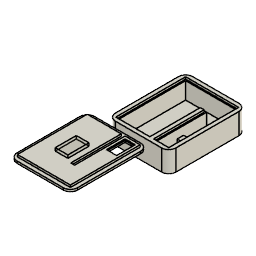
modelo_v2 (Autodesk Fusion 360 design; units mm, degrees)
part number: 2026-04-27-17-29-00-907
Autodesk Fusion 360 part; units mm, degrees
sketch "Boceto1" plane through (0, 0, 0) normal (0, 0, 1) x (1, 0, 0)
  line L0 (115, 170) -> (5, 170)
  arc A0 (5, 170) -> (-10, 155) centre (5, 155) ccw
  line L1 (-10, 155) -> (-10, 5)
  arc A1 (-10, 5) -> (5, -10) centre (5, 5) ccw
  line L2 (5, -10) -> (115, -10)
  arc A2 (115, -10) -> (130, 5) centre (115, 5) ccw
  line L3 (130, 5) -> (130, 155)
  arc A3 (130, 155) -> (115, 170) centre (115, 155) ccw
  line L4 (115, 170) -> (5, 170)
  line L5 (-10, 155) -> (-10, 5)
  line L6 (5, -10) -> (115, -10)
  line L7 (130, 5) -> (130, 155)
  arc A4 (-10, 5) -> (5, -10) centre (5, 5) ccw
  arc A5 (115, -10) -> (130, 5) centre (115, 5) ccw
  arc A6 (5, 170) -> (-10, 155) centre (5, 155) ccw
  arc A7 (130, 155) -> (115, 170) centre (115, 155) ccw
  spline S0 degree 5 poles (115, 0) (115.002, 0) (115.0039, 0) (115.0059, 0) (115.0079, 0) (115.0098, 0) knots 0 0 0 0 0 0 0.001128 0.001128 0.001128 0.001128 0.001128 0.001128
  line L8 (115.0088, 0) -> (115.0108, 0)
  point P0 (0, 160)
  point P1 (130, 170)
  point P2 (-10, 170)
  point P3 (-10, -10)
  dimension "d1" = 160
  dimension "d12" = 180
  dimension "d13" = 140
  dimension "d14" = 15
  dimension "d15" = 15
  dimension "d16" = 15
  constraint horizontal L4
  constraint vertical L5
  constraint horizontal L6
  constraint vertical L7
  constraint coincident P3 L5
  constraint coincident P3 L6
  constraint tangent L5 A4
  constraint tangent L6 A4
  constraint tangent L6 A5
  constraint tangent L7 A5
  constraint equal A4 A5
  constraint coincident P2 L4
  constraint coincident P2 L5
  constraint tangent L4 A6
  constraint tangent L5 A6
  constraint coincident P1 L4
  constraint coincident P1 L7
  constraint tangent L4 A7
  constraint tangent L7 A7
  constraint tangent L3 A3
  constraint tangent L1 A1
  constraint tangent A0 L1
  constraint tangent L0 A3
  constraint tangent L0 A0
  constraint tangent A2 L3
  constraint tangent A1 L2
  constraint tangent L2 A2
  constraint midpoint S0.end L8
  measures "d1" distance of origin P0
  measures "d12" distance of P2 P3
  measures "d13" distance of P1 P2
  measures "d14" radius of A4
  measures "d15" radius of A6
  measures "d16" radius of A7
extrude "Extruir1" add sketch "Boceto1" along normal blind 5 makes body 1
sketch "Boceto2" plane through (0, 0, 5) normal (0, 0, 1) x (-1, 0, 0)
  arc A0 (-130, -155) -> (-115, -170) centre (-115, -155) ccw
  line L0 (-115, -170) -> (-5, -170)
  arc A1 (-5, -170) -> (10, -155) centre (-5, -155) ccw
  line L1 (10, -155) -> (10, -5)
  arc A2 (10, -5) -> (-5, 10) centre (-5, -5) ccw
  line L2 (-5, 10) -> (-115, 10)
  arc A3 (-115, 10) -> (-130, -5) centre (-115, -5) ccw
  line L3 (-130, -5) -> (-130, -155)
  line L4 (0, 0) -> (-120, 0)
  line L5 (-120, 0) -> (-120, -160)
  line L6 (-120, -160) -> (0, -160)
  line L7 (0, -160) -> (0, 0)
  dimension "d20" = 160
  dimension "d21" = 120
  constraint horizontal L4
  constraint vertical L5
  constraint horizontal L6
  constraint vertical L7
  constraint coincident L4.start L7.end
  measures "d20" distance of L4.start L6.end
  measures "d21" distance of L5.end L6.end
extrude "Extruir2" add sketch "Boceto2" along normal blind 80 bodies 1
sketch "Boceto3" plane through (0, 0, 5) normal (0, 0, 1) x (-1, 0, 0)
  line L0 (0, 0) -> (-120, 0)
  line L1 (-120, 0) -> (-120, -160)
  line L2 (-120, -160) -> (0, -160)
  line L3 (0, -160) -> (0, 0)
  line L4 (-90, 0) -> (-75, 0)
  line L5 (-75, 0) -> (-75, -120)
  line L6 (-75, -120) -> (-90, -120)
  line L7 (-90, -120) -> (-90, 0)
  line L8 (-120, -50) -> (-90, -50)
  line L9 (-90, -50) -> (-90, -65)
  line L10 (-90, -65) -> (-120, -65)
  line L11 (-120, -65) -> (-120, -50)
  dimension "d24" = 30
  dimension "d25" = 15
  dimension "d26" = 120
  dimension "d27" = 15
  constraint horizontal L4
  constraint vertical L5
  constraint horizontal L6
  constraint vertical L7
  constraint coincident L0 L4.start
  constraint horizontal L8
  constraint vertical L9
  constraint horizontal L10
  constraint vertical L11
  constraint coincident L7 L9.end
  constraint coincident L1 L8.start
  measures "d24" distance of L9.end L10.end
  measures "d25" distance of L8.start L10.end
  measures "d26" distance of L4.start L6.end
  measures "d27" distance of L5.end L6.end
extrude "Extruir3" add sketch "Boceto3" along normal blind 80 contours L0 L4 L5 L6 L7 L9 bodies 1
sketch "Boceto5" plane through (0, 0, 5) normal (0, 0, 1) x (-1, 0, 0)
  line L0 (-75, 0) -> (-75, -120)
  line L1 (-75, -120) -> (-90, -120)
  line L2 (-90, -120) -> (-90, 0)
  line L3 (-90, 0) -> (-120, 0)
  line L4 (-120, 0) -> (-120, -160)
  line L5 (-120, -160) -> (0, -160)
  line L6 (0, -160) -> (0, 0)
  line L7 (0, 0) -> (-75, 0)
  line L8 (-120, -50) -> (-90, -50)
  line L9 (-90, -50) -> (-90, -65)
  line L10 (-90, -65) -> (-120, -65)
  line L11 (-120, -65) -> (-120, -50)
  dimension "d30" = 15
  dimension "d31" = 30
  constraint horizontal L8
  constraint vertical L9
  constraint horizontal L10
  constraint vertical L11
  constraint coincident L2 L9.end
  constraint coincident L4 L8.start
  measures "d30" distance of L8.start L10.end
  measures "d31" distance of L8.start L8.end
extrude "Extruir4" add sketch "Boceto5" along normal blind 20 contours L2 L4 L8 L9 L10 L11 bodies 1
extrude "Extruir5" cut 1 faces at (85, 40, 85) along direction (0, 0, -1) blind 20 on bodies 1 bodies 1
extrude "Extruir6" cut 1 faces at (85, 40, 65) along direction (0, 0, -1) blind 20 on bodies 1 bodies 1
sketch "Boceto12" plane through (0, 0, 45) normal (0, 0, 1) x (-1, 0, 0)
  line L0 (0, 0) -> (0, -160)
  line L1 (0, -160) -> (-120, -160)
  line L2 (-120, -160) -> (-120, 0)
  line L3 (-120, 0) -> (-90, 0)
  line L4 (-90, 0) -> (-90, -120)
  line L5 (-90, -120) -> (-75, -120)
  line L6 (-75, -120) -> (-75, 0)
  line L7 (-75, 0) -> (0, 0)
  line L8 (-130, -5) -> (-130, -155)
  arc A0 (-130, -155) -> (-115, -170) centre (-115, -155) ccw
  line L9 (-115, -170) -> (-5, -170)
  arc A1 (-5, -170) -> (10, -155) centre (-5, -155) ccw
  line L10 (10, -155) -> (10, -5)
  arc A2 (10, -5) -> (-5, 10) centre (-5, -5) ccw
  line L11 (-5, 10) -> (-115, 10)
  arc A3 (-115, 10) -> (-130, -5) centre (-115, -5) ccw
  line L12 (2, 2) -> (2, -162)
  line L13 (2, -162) -> (-122, -162)
  line L14 (-122, -162) -> (-122, 2)
  line L15 (-122, 2) -> (-88, 2)
  line L16 (-88, 2) -> (-88, -118)
  line L17 (-88, -118) -> (-77, -118)
  line L18 (-77, -118) -> (-77, 2)
  line L19 (-77, 2) -> (2, 2)
  dimension "d41" = -2
extrude "Extruir8" cut sketch "Boceto12" against normal blind 3 contours L12 L13 L14 L15 L16 L17 L18 L19 bodies 1
extrude "Extruir9" add 1 faces at (-10, 105, 15) along direction (-1, 0, 0) blind 2 on bodies 1 bodies 1
extrude "Extruir10" add 1 faces at (41.6667, -10, 30) along direction (0, -1, 0) blind 2 on bodies 1 bodies 1
extrude "Extruir11" add 1 faces at (130, 55, 15) along direction (1, 0, 0) blind 2 on bodies 1 bodies 1
extrude "Extruir12" add 1 faces at (41.6667, 170, 15) along direction (0, 1, 0) blind 2 on bodies 1 bodies 1
move_face "CarasDesfase1" offset 2 1 faces at (-8.3325, 161.8734, 30) on bodies 1
move_face "CarasDesfase2" offset 2 1 faces at (129.175, 159.906, 30) on bodies 1
move_face "CarasDesfase3" offset 2 1 faces at (119.906, -9.175, 30) on bodies 1
move_face "CarasDesfase4" offset 2 1 faces at (4.2863, -9.983, 15) on bodies 1
extrude "Extruir13" add 1 faces at (121.3333, 53.3333, 42) along direction (0, 0, 1) blind 3 on bodies 1 bodies 1
sketch "Boceto14" plane through (0, 0, 45) normal (0, 0, 1) x (-1, 0, 0)
  line L0 (-75, -120) -> (-75, 0)
  line L1 (-75, 0) -> (0, 0)
  line L2 (0, 0) -> (0, -160)
  line L3 (0, -160) -> (-120, -160)
  line L4 (-120, -160) -> (-120, 0)
  line L5 (-120, 0) -> (-90, 0)
  line L6 (-90, 0) -> (-90, -120)
  line L7 (-90, -120) -> (-75, -120)
  line L8 (-5, 12) -> (-115, 12)
  arc A0 (-115, 12) -> (-132, -5) centre (-115, -5) ccw
  line L9 (-132, -5) -> (-132, -155)
  arc A1 (-132, -155) -> (-115, -172) centre (-115, -155) ccw
  line L10 (-115, -172) -> (-5, -172)
  arc A2 (-5, -172) -> (12, -155) centre (-5, -155) ccw
  line L11 (12, -155) -> (12, -5)
  arc A3 (12, -5) -> (-5, 12) centre (-5, -5) ccw
  line L12 (-87, 3) -> (-87, -117)
  line L13 (-87, -117) -> (-78, -117)
  line L14 (-78, -117) -> (-78, 3)
  line L15 (-78, 3) -> (3, 3)
  line L16 (3, 3) -> (3, -163)
  line L17 (3, -163) -> (-123, -163)
  line L18 (-123, -163) -> (-123, 3)
  line L19 (-123, 3) -> (-87, 3)
  dimension "d58" = -3
sketch "Boceto15" plane through (0, 0, 45) normal (0, 0, 1) x (-1, 0, 0)
  line L0 (-75, -120) -> (-75, 0)
  line L1 (-75, 0) -> (0, 0)
  line L2 (0, 0) -> (0, -160)
  line L3 (0, -160) -> (-120, -160)
  line L4 (-120, -160) -> (-120, 0)
  line L5 (-120, 0) -> (-90, 0)
  line L6 (-90, 0) -> (-90, -120)
  line L7 (-90, -120) -> (-75, -120)
  line L8 (-5, 12) -> (-115, 12)
  arc A0 (-115, 12) -> (-132, -5) centre (-115, -5) ccw
  line L9 (-132, -5) -> (-132, -155)
  arc A1 (-132, -155) -> (-115, -172) centre (-115, -155) ccw
  line L10 (-115, -172) -> (-5, -172)
  arc A2 (-5, -172) -> (12, -155) centre (-5, -155) ccw
  line L11 (12, -155) -> (12, -5)
  arc A3 (12, -5) -> (-5, 12) centre (-5, -5) ccw
  line L12 (3, -163) -> (-123, -163)
  line L13 (-123, -163) -> (-123, 3)
  line L14 (-123, 3) -> (-87, 3)
  line L15 (-87, 3) -> (-87, -117)
  line L16 (-87, -117) -> (-78, -117)
  line L17 (-78, -117) -> (-78, 3)
  line L18 (-78, 3) -> (3, 3)
  line L19 (3, 3) -> (3, -163)
  dimension "d61" = -3
extrude "Extruir15" add sketch "Boceto15" along normal blind 10 contours L8 A0 L9 A1 L10 A2 L11 A3 bodies 1
extrude "Extruir16" cut 1 faces at (66, -9, 55) along direction (0, 0, -1) blind 5 on bodies 1 bodies 1
sketch "Boceto17" plane through (0, 0, 50) normal (0, 0, 1) x (-1, 0, 0)
  line L0 (-78, 3) -> (3, 3)
  line L1 (3, 3) -> (3, -163)
  line L2 (3, -163) -> (-123, -163)
  line L3 (-123, -163) -> (-123, 3)
  line L4 (-123, 3) -> (-87, 3)
  line L5 (-87, 3) -> (-87, -117)
  line L6 (-87, -117) -> (-78, -117)
  line L7 (-78, -117) -> (-78, 3)
  arc A0 (12, -5) -> (-5, 12) centre (-5, -5) ccw
  line L8 (-5, 12) -> (-115, 12)
  arc A1 (-115, 12) -> (-132, -5) centre (-115, -5) ccw
  line L9 (-132, -5) -> (-132, -155)
  arc A2 (-132, -155) -> (-115, -172) centre (-115, -155) ccw
  line L10 (-115, -172) -> (-5, -172)
  arc A3 (-5, -172) -> (12, -155) centre (-5, -155) ccw
  line L11 (12, -155) -> (12, -5)
extrude "Extruir17" add sketch "Boceto17" along normal blind 5 bodies 1
sketch "Boceto18" plane through (-12, 0, 0) normal (-1, 0, 0) x (0, -1, 0)
  line L0 (-155, 55) -> (-155, 0)
  line L1 (-155, 0) -> (-5, 0)
  line L2 (-5, 0) -> (-5, 55)
  line L3 (-5, 55) -> (-155, 55)
  line L4 (-155, 50) -> (-5, 50)
  constraint coincident L0 L4.start
  constraint coincident L2 L4.end
  constraint perpendicular L2 L4
split "Dividir1" by curves path "Boceto18" along L4 bodies 1 makes body 2 at (84, 55, 0)
move_body "Desplazar1" bodies 1 to x (1, 0, 0) y (0, 1, 0) z (0, 0, 1) at (0, 0, 55)
sketch "Boceto19" plane through (0, 0, 110) normal (0, 0, 1) x (-1, 0, 0)
  line L0 (-87, -117) -> (-78, -117)
  line L1 (-78, -117) -> (-78, 3)
  line L2 (-78, 3) -> (3, 3)
  line L3 (3, 3) -> (3, -163)
  line L4 (3, -163) -> (-123, -163)
  line L5 (-123, -163) -> (-123, 3)
  line L6 (-123, 3) -> (-87, 3)
  line L7 (-87, 3) -> (-87, -117)
  line L8 (12, -155) -> (12, -5)
  arc A0 (12, -5) -> (-5, 12) centre (-5, -5) ccw
  line L9 (-5, 12) -> (-115, 12)
  arc A1 (-115, 12) -> (-132, -5) centre (-115, -5) ccw
  line L10 (-132, -5) -> (-132, -155)
  arc A2 (-132, -155) -> (-115, -172) centre (-115, -155) ccw
  line L11 (-115, -172) -> (-5, -172)
  arc A3 (-5, -172) -> (12, -155) centre (-5, -155) ccw
extrude "Extruir18" add sketch "Boceto19" against normal blind 10 contours L0 L1 L2 L3 L4 L5 L6 L7 bodies 1
sketch "Boceto20" plane through (0, 0, 5) normal (0, 0, 1) x (-1, 0, 0)
  line L0 (-120, -50) -> (-90, -50)
  line L1 (-90, -50) -> (-90, 0)
  line L2 (-90, 0) -> (-120, 0)
  line L3 (-120, 0) -> (-120, -50)
extrude "Extruir19" cut sketch "Boceto20" along normal blind 105 bodies 1
move_body "Desplazar2" bodies 1 to x (1, 0, 0) y (0, 1, 0) z (0, 0, 1) at (0, 0, -55)
move_body "Desplazar3" bodies 1 to x (1, 0, 0) y (0, 1, 0) z (0, 0, 1) at (0, 0, 65)
sketch "Boceto21" plane through (0, 0, 120) normal (0, 0, 1) x (-1, 0, 0)
  line L0 (-120, 0) -> (-90, 0)
  line L1 (-90, 0) -> (-90, -50)
  line L2 (-90, -50) -> (-120, -50)
  line L3 (-120, -50) -> (-120, 0)
  line L4 (12, -155) -> (12, -5)
  arc A0 (12, -5) -> (-5, 12) centre (-5, -5) ccw
  line L5 (-5, 12) -> (-115, 12)
  arc A1 (-115, 12) -> (-132, -5) centre (-115, -5) ccw
  line L6 (-132, -5) -> (-132, -155)
  arc A2 (-132, -155) -> (-115, -172) centre (-115, -155) ccw
  line L7 (-115, -172) -> (-5, -172)
  arc A3 (-5, -172) -> (12, -155) centre (-5, -155) ccw
  line L8 (-90, -50) -> (-120, -50)
  line L9 (-120, -50) -> (-120, 0)
  line L10 (-120, 0) -> (-90, 0)
  line L11 (-90, 0) -> (-90, -50)
  constraint horizontal L8
  constraint vertical L9
  constraint horizontal L10
  constraint vertical L11
  constraint coincident L0.start L3.end
  constraint coincident L1.end L2.start
extrude "Extruir20" add sketch "Boceto21" along normal blind 5 separate body contours L0 L1 L2 L3 L8 L9 L10 L11 makes body 3
move_body "Desplazar4" bodies 3 to x (1, 0, 0) y (0, 1, 0) z (0, 0, 1) at (0, 0, 25)
sketch "Boceto23" plane through (0, 0, 110) normal (0, 0, -1) x (1, 0, 0)
  line L0 (90, 0) -> (120, 0)
  line L1 (120, 0) -> (120, -50)
  line L2 (120, -50) -> (90, -50)
  line L3 (90, -50) -> (90, 0)
  line L4 (123, 3) -> (87, 3)
  line L5 (87, 3) -> (87, -117)
  line L6 (87, -117) -> (78, -117)
  line L7 (78, -117) -> (78, 3)
  line L8 (78, 3) -> (-3, 3)
  line L9 (-3, 3) -> (-3, -163)
  line L10 (-3, -163) -> (123, -163)
  line L11 (123, -163) -> (123, 3)
  line L12 (93, -3) -> (117, -3)
  line L13 (117, -3) -> (117, -47)
  line L14 (117, -47) -> (93, -47)
  line L15 (93, -47) -> (93, -3)
  dimension "d75" = 3
extrude "Extruir21" add sketch "Boceto23" against normal blind 3 contours L0 L1 L2 L3 bodies 1
extrude "Extruir22" add 1 faces at (110, 16.6667, 150) along direction (0, 0, 1) blind 2 on bodies 3 bodies 3
move_body "Desplazar5" bodies 2 to x (1, 0, 0) y (0, 1, 0) z (0, 0, 1) at (0, 240, 0)
move_body "Desplazar6" bodies 1 to x (1, 0, 0) y (0, -1, 0) z (0, 0, -1) at (0, 166, 200)
named bodies: "Tapa", "Caja", "Cristal"
